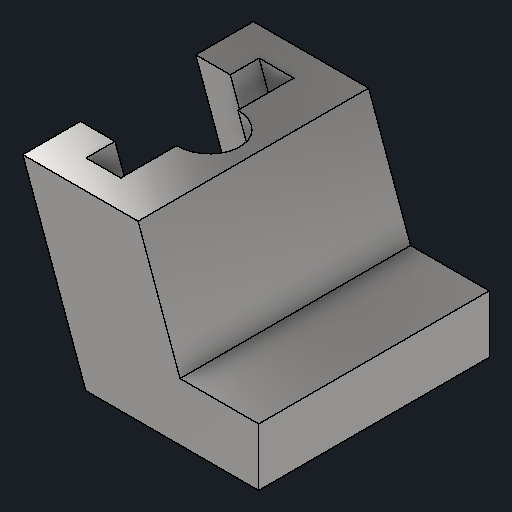
# Autodesk Inventor part: Part1
Saved by Autodesk Inventor 2026.2 (Build 302298000, 298)
## iProperties
Created: 2026-09-23
Part Number: Part1
Material: Steel, Alloy
Document SubType Name: Modeling
Designer: JoshuaEah
Density: 7.73 g/cm^3
Appearance: Semi-Polished
Author: JoshuaEah
Autodesk Inventor part; units mm, degrees
sketch "Sketch1" plane through (0, 0, 0) normal (0, 1, 0) x (-1, 0, 0)
  line L0 (0, 0) -> (-19.05, 0)
  line L1 (-19.05, 0) -> (-19.05, -25.4)
  line L2 (-19.05, -25.4) -> (0, -25.4)
  line L3 (0, -25.4) -> (0, 0)
  line L4 (0, -12.7) -> (-19.05, -12.7) construction
  line L5 (-3.81, -25.4) -> (-3.81, 0)
  line L6 (-12.7, -25.4) -> (-12.7, 0)
  line L7 (-7.62, -25.4) -> (-7.62, 0)
  line L8 (0, -19.05) -> (-3.81, -19.05)
  line L9 (-3.81, -22.225) -> (-7.62, -22.225)
  line L10 (0, -6.35) -> (-3.81, -6.35)
  line L11 (-3.81, -3.175) -> (-7.62, -3.175)
  point P0 (-3.81, -12.7)
  point P1 (-3.81, -6.35)
  point P2 (0, -6.35)
  point P3 (-7.62, -3.175)
  point P4 (-3.81, -3.175)
  dimension "d7" = 25.4
  dimension "d34" = 3.81
  dimension "d57" = 6.35
  dimension "d68" = 3.81
  dimension "d69" = 12.7
  dimension "d70" = 19.05
  dimension "d72" = 12.7
  constraints: 24 end point, 10 point on line, 6 perpendicular, 4 symmetric about line, 3 midpoint, 2 parallel, 1 coincident, 1 horizontal
  measures "d7" distance of L2.end L0.start
  measures "d34" distance between parallel lines of L3 L5
  measures "d57" distance between parallel lines of L1 L6
  measures "d68" distance between parallel lines of L5 L7
  measures "d69" diameter of L8 L4
  measures "d70" diameter of L9 L4
  measures "d72" distance between parallel lines of L3 L6
sketch "Sketch8" plane through (0, 0, 0) normal (0, 0, 1) x (1, 0, 0)
  line L0 (0, 0) -> (-6.9336, 19.05)
  line L1 (0, 0) -> (20.2726, 0) construction
  dimension "d53" = 110
  dimension "d54" = 19.05
  constraints: 4 end point, 1 coincident, 1 equal length, 1 horizontal
  measures "d53" angle of L1 L0
  measures "d54" distance from line of L1 L0.end
sweep "Sweep3" add profiles "Sketch1" path "Sketch8" contours L3 L10 L5 L0 | L5 L11 L7 L0 | L7 L2 L6 L0 | L3 L2 L5 L8 | L9 L5 L2 L7
extrude "Extrusion3" add sketch "Sketch1" along normal blind 6.35 contours L7 L2 L6 L0 | L6 L2 L1 L0
ref_plane "Work Plane6" through (0.6864, 19.05, -25.4) normal (0.342, -0.9397, 0) x (0, 0, 1)
sketch "Sketch9" plane through (0.6864, 19.05, -25.4) normal (0.342, -0.9397, 0) x (0, 0, 1)
  line L0 (3.175, 0) -> (22.225, 0) construction
  point P0 (12.7, 0)
  constraints: 1 midpoint
hole "Hole4" at (0.6864, 19.05, -12.7) direction (0.342, -0.9397, 0) diameter 6.7564 depth 12.7 tip angle 118
ref_plane "Work Plane7" through (-6.9336, 19.05, -25.4) normal (-1, 0, 0) x (0, 0, 1)
ref_plane "Work Plane8" through (0, 0, -6.35) normal (0, -1, 0) x (1, 0, 0)
ref_plane "Work Plane9" through (-6.9336, 19.05, -25.4) normal (-0.342, 0.9397, 0) x (0, 0, 1)
ref_plane "Work Plane10" through (10.3888, 6.35, -6.35) normal (0.342, -0.9397, 0) x (0, 0, -1)
equation "\"d34\" = slotWidth"
equation "\"d68\" = d34"
equation "\"slopeAngle\" = 70deg"
equation "\"slotWidth\" = 3.81"
body "Solid4"
